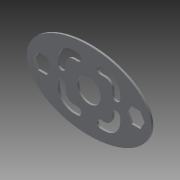
# Autodesk Inventor part: HW 6 Part 3
Saved by Autodesk Inventor 2015 SP1 (Build 190203100, 203)
## iProperties
Created: 2016-02-10
Part Number: HW 6 Part 3
Material: Generic
Document SubType Name: Modeling
Designer: melissa.roth
Density: 1 g/cm^3
Appearance: Default
Author: melissa.roth
Autodesk Inventor part; units mm, degrees
ref_plane "YZ Plane" through (0, 0, 0) normal (1, 0, 0) x (0, 1, 0)
ref_plane "XZ Plane" through (0, 0, 0) normal (0, 1, 0) x (-1, 0, 0)
ref_plane "XY Plane" through (0, 0, 0) normal (0, 0, 1) x (1, 0, 0)
sketch "Sketch1" plane through (0, 0, 0) normal (0, 0, 1) x (1, 0, 0)
  ellipse E0 centre (0, 0) end of major axis (101.6, 0) minor radius 63.5
  line L0 (-90.6584, 0) -> (-83.4914, 12.7)
  line L1 (-83.4914, 12.7) -> (-68.9086, 12.7)
  line L2 (-68.9086, 12.7) -> (-61.7416, 0)
  line L3 (-61.7416, 0) -> (-68.9086, -12.7)
  line L4 (-68.9086, -12.7) -> (-83.4914, -12.7)
  line L5 (-83.4914, -12.7) -> (-90.6584, 0)
  line L6 (90.6584, 0) -> (83.4914, 12.7)
  line L7 (83.4914, 12.7) -> (68.9086, 12.7)
  line L8 (68.9086, 12.7) -> (61.7416, 0)
  line L9 (61.7416, 0) -> (68.9086, -12.7)
  line L10 (68.9086, -12.7) -> (83.4914, -12.7)
  line L11 (83.4914, -12.7) -> (90.6584, 0)
  line L12 (0, 0) -> (0, -14.2875)
  arc A0 (19.05, -31.75) -> (19.05, -44.45) centre (19.05, -38.1) ccw
  line L13 (25.4, -44.45) -> (19.05, -44.45)
  line L14 (25.4, -31.75) -> (19.05, -31.75)
  line L15 (38.1, -19.05) -> (38.1, -12.7)
  arc A1 (25.4, -31.75) -> (38.1, -19.05) centre (25.4, -19.05) ccw
  line L16 (50.8, -19.05) -> (50.8, -12.7)
  arc A2 (25.4, -44.45) -> (50.8, -19.05) centre (25.4, -19.05) ccw
  arc A3 (50.8, -12.7) -> (38.1, -12.7) centre (44.45, -12.7) ccw
  circle A4 centre (0, 0) radius 19.05
  line L17 (0, 19.05) -> (0, -19.05)
  line L18 (-19.05, 0) -> (19.05, 0)
  line L19 (-38.1, -19.05) -> (-38.1, -12.7)
  line L20 (-50.8, -19.05) -> (-50.8, -12.7)
  arc A5 (-38.1, -12.7) -> (-50.8, -12.7) centre (-44.45, -12.7) ccw
  arc A6 (-38.1, -19.05) -> (-25.4, -31.75) centre (-25.4, -19.05) ccw
  arc A7 (-50.8, -19.05) -> (-25.4, -44.45) centre (-25.4, -19.05) ccw
  line L21 (-25.4, -31.75) -> (-19.05, -31.75)
  line L22 (-25.4, -44.45) -> (-19.05, -44.45)
  arc A8 (-19.05, -44.45) -> (-19.05, -31.75) centre (-19.05, -38.1) ccw
  line L23 (38.1, 19.05) -> (38.1, 12.7)
  line L24 (50.8, 19.05) -> (50.8, 12.7)
  arc A9 (38.1, 12.7) -> (50.8, 12.7) centre (44.45, 12.7) ccw
  arc A10 (38.1, 19.05) -> (25.4, 31.75) centre (25.4, 19.05) ccw
  arc A11 (50.8, 19.05) -> (25.4, 44.45) centre (25.4, 19.05) ccw
  line L25 (25.4, 31.75) -> (19.05, 31.75)
  line L26 (25.4, 44.45) -> (19.05, 44.45)
  arc A12 (19.05, 44.45) -> (19.05, 31.75) centre (19.05, 38.1) ccw
  arc A13 (-25.4, 31.75) -> (-38.1, 19.05) centre (-25.4, 19.05) ccw
  arc A14 (-25.4, 44.45) -> (-50.8, 19.05) centre (-25.4, 19.05) ccw
  line L27 (-25.4, 31.75) -> (-19.05, 31.75)
  line L28 (-38.1, 19.05) -> (-38.1, 12.7)
  arc A15 (-50.8, 12.7) -> (-38.1, 12.7) centre (-44.45, 12.7) ccw
  line L29 (-50.8, 19.05) -> (-50.8, 12.7)
  arc A16 (-19.05, 31.75) -> (-19.05, 44.45) centre (-19.05, 38.1) ccw
  line L30 (-25.4, 44.45) -> (-19.05, 44.45)
  point P0 (65.3251, -6.35)
  dimension "d0" = 101.6
  dimension "d56" = 63.5
  dimension "d3" = 25.4
  dimension "d44" = 25.4
  dimension "d45" = 50.8
  dimension "d47" = 6.35
  dimension "d50" = 25.4
  dimension "d51" = 19.05
  dimension "d52" = 6.35
  dimension "d53" = 6.35
  dimension "d54" = 6.35
  dimension "d55" = 38.1
  constraints: 62 end point, 36 point on circle, 36 symmetric about line, 17 centre point, 8 equal length, 7 coincident, 6 tangent, 3 horizontal, 3 midpoint, 2 vertical, 1 parallel, 24 other
  measures "d3" distance between parallel lines of L4 L1
  measures "d44" diameter of A1
  measures "d45" diameter of A2
  measures "d47" radius of A3
  measures "d50" horizontal distance of A2.centre point (0, 0)
  measures "d51" vertical distance of A2.centre point (0, 0)
  measures "d52" distance of L13.start L13.end
  measures "d53" horizontal distance of A2.centre A0.centre
  measures "d54" vertical distance of A1.centre A3.centre
  measures "d55" diameter of A4
extrude "Extrusion2" add sketch "Sketch1" along normal blind 3.175
body "Solid2"
